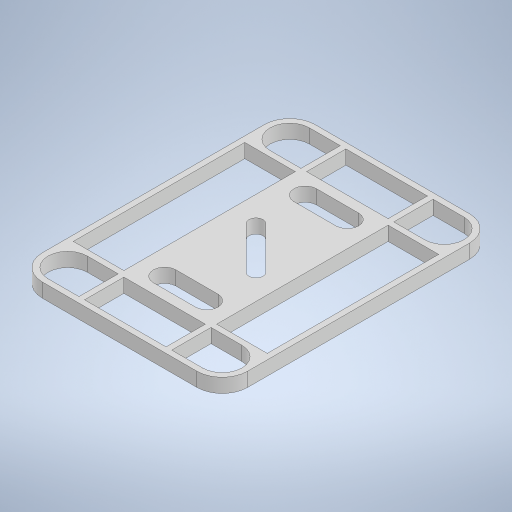
# Autodesk Inventor part: Stand Brace
Saved by Autodesk Inventor 2024.1 (Build 281209000, 209)
## iProperties
Created: 2024-01-03
Part Number: Stand Brace
Material: Generic
Document SubType Name: Modeling
Designer: ryanm
Density: 1 g/cm^3
Appearance: Default
Author: ryanm
Autodesk Inventor part; units mm, degrees
ref_plane "YZ Plane" through (0, 0, 0) normal (1, 0, 0) x (0, 1, 0)
ref_plane "XZ Plane" through (0, 0, 0) normal (0, 1, 0) x (-1, 0, 0)
ref_plane "XY Plane" through (0, 0, 0) normal (0, 0, 1) x (1, 0, 0)
sketch "Sketch1" plane through (0, 0, 0) normal (0, 1, 0) x (-1, 0, 0)
  line L0 (36.5, 39.5) -> (36.5, 0)
  arc A0 (36.5, 39.5) -> (27.5, 48.5) centre (27.5, 39.5) ccw
  line L1 (27.5, 48.5) -> (0, 48.5)
  line L2 (0, 48.5) -> (0, 0) construction
  arc A1 (27.5, 32.5) -> (27.5, 46.5) centre (27.5, 39.5) ccw
  line L3 (27.5, 46.5) -> (16.5, 46.5)
  line L4 (16.5, 32.5) -> (27.5, 32.5)
  line L5 (16.5, 32.5) -> (16.5, 46.5)
  line L6 (16.5, 30.5) -> (16.5, 0)
  line L7 (14.5, 32.5) -> (0, 32.5)
  line L8 (14.5, 46.5) -> (0, 46.5)
  line L9 (14.5, 46.5) -> (14.5, 32.5)
  line L10 (14.5, 30.5) -> (14.5, 0)
  line L11 (34.5, 30.5) -> (16.5, 30.5)
  line L12 (14.5, 30.5) -> (0, 30.5)
  line L13 (34.5, 30.5) -> (34.5, -1)
  line L14 (36.5, 0) -> (0, 0) construction
  line L15 (-36.5, 39.5) -> (-36.5, 0)
  line L16 (-27.5, 48.5) -> (0, 48.5)
  arc A2 (-27.5, 48.5) -> (-36.5, 39.5) centre (-27.5, 39.5) ccw
  arc A3 (-27.5, 46.5) -> (-27.5, 32.5) centre (-27.5, 39.5) ccw
  line L17 (-27.5, 46.5) -> (-16.5, 46.5)
  line L18 (-16.5, 32.5) -> (-27.5, 32.5)
  line L19 (-16.5, 32.5) -> (-16.5, 46.5)
  line L20 (-16.5, 30.5) -> (-16.5, 0)
  line L21 (-14.5, 32.5) -> (0, 32.5)
  line L22 (-14.5, 46.5) -> (0, 46.5)
  line L23 (-14.5, 46.5) -> (-14.5, 32.5)
  line L24 (-14.5, 30.5) -> (-14.5, 0)
  line L25 (-34.5, 30.5) -> (-16.5, 30.5)
  line L26 (-14.5, 30.5) -> (0, 30.5)
  line L27 (-34.5, 30.5) -> (-34.5, -1)
  line L28 (36.5, -39.5) -> (36.5, 0)
  line L29 (27.5, -48.5) -> (0, -48.5)
  arc A4 (27.5, -48.5) -> (36.5, -39.5) centre (27.5, -39.5) ccw
  line L30 (0, -48.5) -> (0, 0) construction
  arc A5 (27.5, -46.5) -> (27.5, -32.5) centre (27.5, -39.5) ccw
  line L31 (27.5, -46.5) -> (16.5, -46.5)
  line L32 (16.5, -32.5) -> (27.5, -32.5)
  line L33 (16.5, -32.5) -> (16.5, -46.5)
  line L34 (16.5, -30.5) -> (16.5, 0)
  line L35 (14.5, -32.5) -> (0, -32.5)
  line L36 (14.5, -46.5) -> (0, -46.5)
  line L37 (14.5, -46.5) -> (14.5, -32.5)
  line L38 (14.5, -30.5) -> (14.5, 0)
  line L39 (34.5, -30.5) -> (16.5, -30.5)
  line L40 (14.5, -30.5) -> (0, -30.5)
  line L41 (34.5, -30.5) -> (34.5, -1)
  line L42 (-36.5, -39.5) -> (-36.5, 0)
  line L43 (-16.5, -30.5) -> (-16.5, 0)
  line L44 (-14.5, -30.5) -> (-14.5, 0)
  line L45 (-34.5, -30.5) -> (-34.5, -1)
  line L46 (-34.5, -30.5) -> (-16.5, -30.5)
  line L47 (-16.5, -32.5) -> (-27.5, -32.5)
  arc A6 (-27.5, -32.5) -> (-27.5, -46.5) centre (-27.5, -39.5) ccw
  arc A7 (-36.5, -39.5) -> (-27.5, -48.5) centre (-27.5, -39.5) ccw
  line L48 (-14.5, -30.5) -> (0, -30.5)
  line L49 (-14.5, -32.5) -> (0, -32.5)
  line L50 (-16.5, -32.5) -> (-16.5, -46.5)
  line L51 (-14.5, -46.5) -> (-14.5, -32.5)
  line L52 (-27.5, -48.5) -> (0, -48.5)
  line L53 (-27.5, -46.5) -> (-16.5, -46.5)
  line L54 (-14.5, -46.5) -> (0, -46.5)
  point P0 (34.5, 39.5)
  point P1 (-34.5, 39.5)
  point P2 (34.5, -39.5)
  point P3 (-34.5, -39.5)
  dimension "d42" = 14
  dimension "d43" = 11
  dimension "d45" = 2
  dimension "d46" = 2
  dimension "d47" = 48.5
  dimension "d48" = 27.5
  dimension "d49" = 2
  dimension "d50" = 2
  dimension "d51" = 2
  dimension "d53" = 31.5
  constraints: 110 end point, 51 symmetric about line, 17 point on circle, 8 centre point, 8 point on line, 6 coincident, 6 horizontal alignment, 5 perpendicular, 5 vertical alignment, 4 vertical, 3 tangent, 2 horizontal, 1 parallel, 6 other
  measures "d42" diameter of A1
  measures "d43" distance of L3.start L3.end
  measures "d45" distance between parallel lines of L1 L3
  measures "d46" distance from line of L0 point (34.5, 39.5)
  measures "d47" distance of L2.start L2.end
  measures "d48" distance from line of L2 A0.centre
  measures "d49" distance between parallel lines of L9 L5
  measures "d50" distance between parallel lines of L11 L4
  measures "d51" distance between parallel lines of L0 L13
  measures "d53" distance from line of L13.end L11
extrude "Extrusion1" add sketch "Sketch1" along normal blind 5
sketch "Sketch8" plane through (0, 5, 0) normal (0, 1, 0) x (1, 0, 0)
  line L0 (-27.5, -48.5) -> (27.5, -48.5) projected
  arc A0 (27.5, -48.5) -> (36.5, -39.5) centre (27.5, -39.5) ccw projected
  line L1 (36.5, -39.5) -> (36.5, 39.5) projected
  arc A1 (36.5, 39.5) -> (27.5, 48.5) centre (27.5, 39.5) ccw projected
  line L2 (27.5, 48.5) -> (-27.5, 48.5) projected
  arc A2 (-27.5, 48.5) -> (-36.5, 39.5) centre (-27.5, 39.5) ccw projected
  line L3 (-36.5, 39.5) -> (-36.5, -39.5) projected
  arc A3 (-36.5, -39.5) -> (-27.5, -48.5) centre (-27.5, -39.5) ccw projected
  line L4 (16.5, 32.5) -> (16.5, 46.5) projected
  line L5 (16.5, 46.5) -> (27.5, 46.5) projected
  arc A4 (27.5, 32.5) -> (27.5, 46.5) centre (27.5, 39.5) ccw projected
  line L6 (27.5, 32.5) -> (16.5, 32.5) projected
  line L7 (14.5, 46.5) -> (14.5, 32.5) projected
  line L8 (14.5, 32.5) -> (-14.5, 32.5) projected
  line L9 (-14.5, 32.5) -> (-14.5, 46.5) projected
  line L10 (-14.5, 46.5) -> (14.5, 46.5) projected
  line L11 (-27.5, 46.5) -> (-16.5, 46.5) projected
  line L12 (-16.5, 46.5) -> (-16.5, 32.5) projected
  line L13 (-16.5, 32.5) -> (-27.5, 32.5) projected
  arc A5 (-27.5, 46.5) -> (-27.5, 32.5) centre (-27.5, 39.5) ccw projected
  line L14 (27.5, -46.5) -> (16.5, -46.5) projected
  line L15 (16.5, -46.5) -> (16.5, -32.5) projected
  line L16 (16.5, -32.5) -> (27.5, -32.5) projected
  arc A6 (27.5, -46.5) -> (27.5, -32.5) centre (27.5, -39.5) ccw projected
  line L17 (34.5, -30.5) -> (16.5, -30.5) projected
  line L18 (16.5, -30.5) -> (16.5, 30.5) projected
  line L19 (16.5, 30.5) -> (34.5, 30.5) projected
  line L20 (34.5, 30.5) -> (34.5, -30.5) projected
  line L21 (14.5, -30.5) -> (-14.5, -30.5) projected
  line L22 (-14.5, -30.5) -> (-14.5, 30.5) projected
  line L23 (-14.5, 30.5) -> (14.5, 30.5) projected
  line L24 (14.5, 30.5) -> (14.5, -30.5) projected
  line L25 (-14.5, -46.5) -> (-14.5, -32.5) projected
  line L26 (-14.5, -32.5) -> (14.5, -32.5) projected
  line L27 (14.5, -32.5) -> (14.5, -46.5) projected
  line L28 (14.5, -46.5) -> (-14.5, -46.5) projected
  line L29 (-34.5, -30.5) -> (-34.5, 30.5) projected
  line L30 (-34.5, 30.5) -> (-16.5, 30.5) projected
  line L31 (-16.5, 30.5) -> (-16.5, -30.5) projected
  line L32 (-16.5, -30.5) -> (-34.5, -30.5) projected
  line L33 (-16.5, -32.5) -> (-16.5, -46.5) projected
  line L34 (-16.5, -46.5) -> (-27.5, -46.5) projected
  arc A7 (-27.5, -32.5) -> (-27.5, -46.5) centre (-27.5, -39.5) ccw projected
  line L35 (-27.5, -32.5) -> (-16.5, -32.5) projected
  point P0 (0, 0)
extrude "Extrusion7" add sketch "Sketch8" against normal up to surface (5 mm away) contours L21 L22 L23 L24
sketch "Sketch9" plane through (0, 5, 0) normal (0, 1, 0) x (1, 0, 0)
  line L0 (-7.5, 25) -> (7.5, 25) construction
  line L1 (-7.5, 21) -> (7.5, 21)
  line L2 (7.5, 29) -> (-7.5, 29)
  arc A0 (-7.5, 29) -> (-7.5, 21) centre (-7.5, 25) ccw
  arc A1 (7.5, 21) -> (7.5, 29) centre (7.5, 25) ccw
  line L3 (-7.5, -25) -> (7.5, -25) construction
  line L4 (-7.5, -29) -> (7.5, -29)
  line L5 (7.5, -21) -> (-7.5, -21)
  arc A2 (-7.5, -21) -> (-7.5, -29) centre (-7.5, -25) ccw
  arc A3 (7.5, -29) -> (7.5, -21) centre (7.5, -25) ccw
  line L6 (-7.5, 7.5) -> (7.5, -7.5) construction
  line L7 (-9.2678, 5.7322) -> (5.7322, -9.2678)
  line L8 (9.2678, -5.7322) -> (-5.7322, 9.2678)
  arc A4 (-5.7322, 9.2678) -> (-9.2678, 5.7322) centre (-7.5, 7.5) ccw
  arc A5 (5.7322, -9.2678) -> (9.2678, -5.7322) centre (7.5, -7.5) ccw
  point P0 (0, 0)
  point P1 (0, 25)
  point P2 (0, -25)
  point P3 (0, 0)
  dimension "d67" = 8
  dimension "d68" = 8
  dimension "d69" = 5
  dimension "d70" = 15
  dimension "d71" = 15
  dimension "d72" = 15
  dimension "d73" = 15
  dimension "d74" = 25
  dimension "d75" = 25
  constraints: 24 end point, 12 point on circle, 12 tangent, 6 centre point, 4 parallel, 3 midpoint, 2 coincident, 2 vertical alignment, 1 horizontal
  measures "d67" diameter of A1
  measures "d68" diameter of A3
  measures "d69" diameter of A5
  measures "d70" distance of L0.start L0.end
  measures "d71" distance of L3.start L3.end
  measures "d72" horizontal distance of L6.start L6.end
  measures "d73" horizontal distance of L6.start L6.end
  measures "d74" distance of point (0, 0) point (0, 25)
  measures "d75" distance of point (0, -25) point (0, 0)
extrude "Extrusion8" cut sketch "Sketch9" against normal through all
equation "\"d50\" = d49"
equation "\"d51\" = d46"
equation "\"d73\" = d72"
equation "\"d75\" = d74"
equation "\"d21\" = d20"
equation "\"d33\" = d32"
equation "\"d20\" = 2"
equation "\"d32\" = 2"
body "Solid1"
